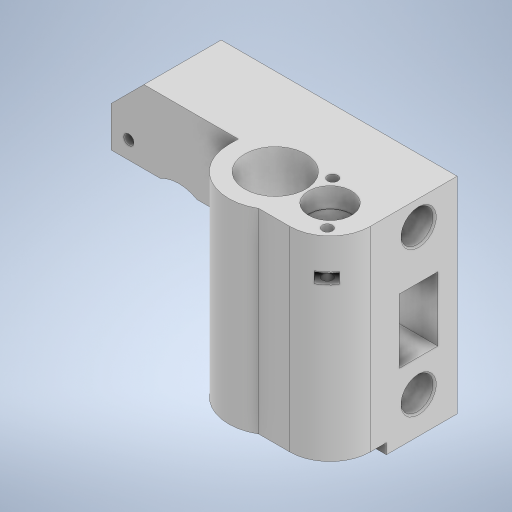
# Autodesk Inventor part: X-End-motor v0.3
Saved by Autodesk Inventor 2023 (Build 270158000, 158)
## iProperties
Created: 2023-07-24
Part Number: X-End-motor v0.3
Material: Generic
Document SubType Name: Modeling
Designer: Parker
Density: 1 g/cm^3
Appearance: Default
Author: Parker
Autodesk Inventor part; units mm, degrees
ref_plane "TopRodPlane" through (0, 22.5, 0) normal (0, 1, 0) x (-1, 0, 0)
ref_plane "BottomRodPlane" through (0, -22.5, 0) normal (0, 1, 0) x (-1, 0, 0)
ref_plane "Work Plane3" through (0, 0, 15) normal (0, 0, 1) x (1, 0, 0)
ref_plane "Work Plane4" through (-17, 0, 0) normal (1, 0, 0) x (0, 1, 0)
ref_plane "MotorZPlane" through (0, -2.5, 0) normal (0, 1, 0) x (-1, 0, 0)
ref_plane "Work Plane6" through (-50, 0, 0) normal (1, 0, 0) x (0, 1, 0)
ref_plane "RearClearancePlane" through (0, 0, -14) normal (0, 0, 1) x (1, 0, 0)
ref_plane "RightClearancePlane" through (14.5, 0, 0) normal (1, 0, 0) x (0, 1, 0)
sketch "Z-Template" plane through (0, 0, 0) normal (0, 1, 0) x (-1, 0, 0)
  circle A0 centre (17, 15) radius 9.5
  circle A1 centre (0, 15) radius 4.5
  circle A2 centre (17, 15) radius 14.5
  line L0 (87.7, 0) -> (-29.2, 0) construction
  line L1 (-29.2, -14) -> (87.7, -14) construction
  circle A3 centre (0, 15) radius 12.5
  line L2 (-14.5, -22.7) -> (-14.5, 38.2) construction
  line L3 (71, 12) -> (-12.5, 12)
  line L4 (-12.5, 12) -> (-12.5, -12)
  line L5 (-12.5, -12) -> (71, -12)
  line L6 (71, -12) -> (71, 12)
  line L7 (71, 12) -> (-12.5, -12) construction
  line L8 (-12.5, 12) -> (71, -12) construction
  line L9 (50, 38.2) -> (50, -22.7) construction
  point P0 (0, 0)
  point P1 (29.25, 0)
  dimension "d7" = 19
  dimension "d8" = 9
  dimension "d9" = 5
  dimension "d11" = 25
  dimension "d12" = 2
  dimension "d13" = 2
  dimension "d14" = 21
  constraints: 12 end point, 4 centre point, 3 coincident, 3 midpoint, 2 parallel, 1 horizontal, 1 perpendicular
  measures "d7" diameter of A0
  measures "d8" diameter of A1
  measures "d9" radial gap between concentric circles of A0 A2
  measures "d11" diameter of A3
  measures "d12" distance between parallel lines of L2 L4
  measures "d13" distance between parallel lines of L1 L5
  measures "d14" distance between parallel lines of L6 L9
ref_plane "TopPlane" through (0, 30, 0) normal (0, 1, 0) x (-1, 0, 0)
sketch "X-Template" plane through (0, 0, 0) normal (0, 0, 1) x (1, 0, 0)
  line L0 (-71, 18.5) -> (-29, 18.5)
  line L1 (-29, 18.5) -> (-29, -23.5)
  line L2 (-29, -23.5) -> (-71, -23.5)
  line L3 (-71, -23.5) -> (-71, 18.5)
  line L4 (-71, 18.5) -> (-29, -23.5) construction
  line L5 (-29, 18.5) -> (-71, -23.5) construction
  line L6 (-65.5, 13) -> (-34.5, 13) construction
  line L7 (-34.5, 13) -> (-34.5, -18) construction
  line L8 (-34.5, -18) -> (-65.5, -18) construction
  line L9 (-65.5, -18) -> (-65.5, 13) construction
  line L10 (-65.5, 13) -> (-34.5, -18) construction
  line L11 (-34.5, 13) -> (-65.5, -18) construction
  circle A0 centre (-65.5, 13) radius 1.6
  circle A1 centre (-34.5, 13) radius 1.6
  circle A2 centre (-34.5, -18) radius 1.6
  circle A3 centre (-65.5, -18) radius 1.6
  circle A4 centre (-50, -2.5) radius 11.5
  line L12 (-87.7, 22.5) -> (29.2, 22.5) projected
  line L13 (-87.7, -22.5) -> (29.2, -22.5) projected
  line L14 (14.5, 42.75) -> (14.5, -46.5) projected
  line L15 (-87.7, 30) -> (29.2, 30) projected
  line L16 (-19, 15) -> (12.5, 15)
  line L17 (12.5, 15) -> (12.5, 30)
  line L18 (12.5, 30) -> (-19, 30)
  line L19 (-19, 30) -> (-19, 15)
  line L20 (-19, 15) -> (12.5, 30) construction
  line L21 (12.5, 15) -> (-19, 30) construction
  line L22 (-19, -30) -> (12.5, -30)
  line L23 (-19, -15) -> (-19, -30)
  line L24 (12.5, -15) -> (-19, -15)
  line L25 (12.5, -30) -> (12.5, -15)
  line L26 (-17, -46.5) -> (-17, 42.75) projected
  line L27 (-7.5, -30.5) -> (-26.5, -30.5)
  line L28 (-26.5, -30.5) -> (-26.5, 30) construction
  line L29 (-26.5, 30) -> (-7.5, 30)
  line L30 (-7.5, 30) -> (-7.5, -30.5) construction
  line L31 (-7.5, -30.5) -> (-26.5, 30) construction
  line L32 (-26.5, -30.5) -> (-7.5, 30) construction
  line L33 (-31.5, 30) -> (-2.5, 30)
  line L34 (-2.5, 30) -> (-2.5, -30.5)
  line L35 (-2.5, -30.5) -> (-31.5, -30.5)
  line L36 (-31.5, -30.5) -> (-31.5, 30)
  line L37 (-31.5, 30) -> (-2.5, -30.5) construction
  line L38 (-2.5, 30) -> (-31.5, -30.5) construction
  point P0 (0, 0)
  point P1 (-3.25, 22.5)
  point P2 (-17, -0.25)
  dimension "d16" = 42
  dimension "d17" = 42
  dimension "d18" = 31
  dimension "d19" = 31
  dimension "d20" = 3.2
  dimension "d21" = 3.2
  dimension "d22" = 3.2
  dimension "d23" = 3.2
  dimension "d24" = 23
  dimension "d25" = 0
  dimension "d26" = 2
  dimension "d27" = 31.5
  dimension "d30" = 45
  dimension "d35" = 60.5
  dimension "d36" = 19
  dimension "d37" = 29
  constraints: 68 end point, 10 midpoint, 10 parallel, 5 centre point, 5 coincident, 5 horizontal, 5 perpendicular, 4 point on line, 1 vertical, 8 other
  measures "d16" distance of L1.end L2.end
  measures "d17" distance of L0.end L1.end
  measures "d18" distance of L7.end L8.end
  measures "d19" distance of L6.end L7.end
  measures "d20" diameter of A0
  measures "d21" diameter of A1
  measures "d22" diameter of A2
  measures "d23" diameter of A3
  measures "d24" diameter of A4
  measures "d25" distance between parallel lines of L15 L18
  measures "d26" distance between parallel lines of L14 L17
  measures "d27" distance between parallel lines of L17 L19
  measures "d30" distance of L16.start L22.start
  measures "d35" distance of L27.end L28.end
  measures "d36" distance between parallel lines of L30 L28
  measures "d37" distance of L34.end L35.end
sketch "Y-Template" plane through (0, 0, 0) normal (1, 0, 0) x (0, 1, 0)
  line L0 (-2.5, 38.2) -> (-2.5, -22.7) construction
  circle A0 centre (22.5, 0) radius 5
  circle A1 centre (-22.5, 0) radius 5
  line L1 (-46.5, 0) -> (42.75, 0) construction
  line L2 (-46.5, 0) -> (42.75, 0) projected
  line L3 (7.5, 6) -> (-12.5, 6)
  line L4 (-12.5, 6) -> (-12.5, -6)
  line L5 (-12.5, -6) -> (7.5, -6)
  line L6 (7.5, -6) -> (7.5, 6)
  line L7 (7.5, 6) -> (-12.5, -6) construction
  line L8 (-12.5, 6) -> (7.5, -6) construction
  line L9 (30, 38.2) -> (30, -22.7) construction
  circle A2 centre (22.5, 0) radius 7.5
  circle A3 centre (-22.5, 0) radius 7.5
  line L10 (-46.5, -14) -> (42.75, -14) projected
  line L11 (-33.75, 29.5) -> (-33.75, -14)
  line L12 (-33.75, -14) -> (30, -14)
  line L13 (30, -14) -> (30, 29.5)
  line L14 (-33.75, 29.5) -> (30, 29.5)
  line L15 (-46.5, 15) -> (42.75, 15) projected
  point P0 (0, 0)
  point P1 (-2.5, 0)
  dimension "d38" = 10
  dimension "d39" = 10
  dimension "d40" = 20
  dimension "d41" = 12
  dimension "d42" = 2.5
  dimension "d43" = 2.5
  dimension "d44" = 11.25
  dimension "d45" = 0
  dimension "d46" = 14.5
  constraints: 20 end point, 4 centre point, 3 point on line, 2 coincident, 2 horizontal, 2 midpoint, 2 parallel, 2 perpendicular, 1 vertical, 3 other
  measures "d38" diameter of A0
  measures "d39" diameter of A1
  measures "d40" distance of L5.end L4.end
  measures "d41" distance of L4.end L3.end
  measures "d42" radial gap between concentric circles of A0 A2
  measures "d43" radial gap between concentric circles of A1 A3
  measures "d44" distance from line of point (-22.5, 0) L11
  measures "d45" distance between parallel lines of L10 L12
  measures "d46" distance between parallel lines of L15 L14
sketch "Z-Drawing" plane through (0, 0, 0) normal (0, 1, 0) x (-1, 0, 0)
  line L0 (71, 12) -> (-12.5, 12) construction
  line L1 (71, -12) -> (71, 12) construction
  line L2 (-12.5, -12) -> (71, -12) construction
  line L3 (-12.5, 12) -> (-12.5, -12) construction
  circle A0 centre (0, 15) radius 12.5 construction
  circle A1 centre (17, 15) radius 14.5 construction
  circle A2 centre (17, 15) radius 9.5 construction
  circle A3 centre (0, 15) radius 4.5 construction
  line L4 (-12.5, 12) -> (-12.5, 15)
  line L5 (0, 27.5) -> (9.6515, 27.5)
  line L6 (31.5, 15) -> (31.5, 12)
  arc A4 (31.5, 15) -> (9.6515, 27.5) centre (17, 15) ccw
  line L7 (31.5, 12) -> (71, 12)
  circle A5 centre (17, 15) radius 9.5
  circle A6 centre (0, 15) radius 4.5
  arc A7 (0, 27.5) -> (-12.5, 15) centre (0, 15) ccw
  line L8 (71, 12) -> (71, -12)
  line L9 (71, -12) -> (-12.5, -12)
  line L10 (-12.5, -12) -> (-12.5, 12)
  point P0 (0, 0)
  dimension "d47" = 19
  dimension "d48" = 9
  dimension "d49" = 0
  constraints: 14 end point, 8 point on circle, 4 centre point, 4 coincident, 3 perpendicular, 2 collinear, 2 tangent, 1 horizontal, 1 point on line
  measures "d47" diameter of A5
  measures "d48" diameter of A6
  measures "d49" horizontal distance of A0.centre L5.start
extrude "Extrusion1" add sketch "Z-Drawing" against normal blind 60.5 from surface at 30
sketch "Y-Sketch" plane through (0, 0, 0) normal (1, 0, 0) x (0, 1, 0)
  circle A0 centre (22.5, 0) radius 5 projected
  line L0 (-12.5, 6) -> (-12.5, -6) projected
  line L1 (-12.5, -6) -> (7.5, -6) projected
  line L2 (7.5, -6) -> (7.5, 6) projected
  line L3 (7.5, 6) -> (-12.5, 6) projected
  circle A1 centre (-22.5, 0) radius 5 projected
  point P0 (0, 0)
extrude "Extrusion2" cut sketch "Y-Sketch" along normal through all both and the other way through all contours L3 L2 L1 L0
extrude "Extrusion3" cut sketch "Y-Sketch" against normal blind 26.5 from surface at 12.5 contours A0 | A1
sketch "X-Sketch" plane through (0, 0, 0) normal (0, 0, 1) x (1, 0, 0)
  circle A0 centre (-65.5, 13) radius 1.6 projected
  circle A1 centre (-34.5, 13) radius 1.6 projected
  circle A2 centre (-34.5, -18) radius 1.6 projected
  circle A3 centre (-50, -2.5) radius 11.5 projected
  line L0 (-71, -30.5) -> (12.5, -30.5) projected
  line L1 (-71, -30.5) -> (-71, 30) projected
  line L2 (-71, 30) -> (12.5, 30) projected
  line L3 (12.5, -30.5) -> (12.5, 30) projected
  line L4 (-71, 7.5) -> (12.5, 7.5) projected
  line L5 (-71, -12.5) -> (-71, 7.5) projected
  line L6 (12.5, -12.5) -> (-71, -12.5) projected
  line L7 (12.5, 7.5) -> (12.5, -12.5) projected
  line L8 (-71, 18.5) -> (-29, 18.5) projected
  line L9 (-29, 18.5) -> (-29, -23.5) projected
  line L10 (-29, -23.5) -> (-71, -23.5) projected
  line L11 (-38.5, 7.5) -> (-38.5, -30.5)
  point P0 (0, 0)
  point P1 (-44.3211, 7.5)
  point P2 (-55.6789, 7.5)
  dimension "d56" = 11.5
  constraints: 2 end point, 2 point on line, 1 perpendicular
  measures "d56" distance from line of A3.centre L11
extrude "Extrusion4" cut sketch "X-Sketch" along normal through all both and the other way through all contours A3 L6 L4 | L11 L6 A3 | A3 L4 L11 | L4 A3 | L6 L11 L10 L1 A3 | A3 L6 | A3 L6 L1 L4 | L11 L0 L1 L10
hole "Hole1" at (-65.5, 13, 0) at (-34.5, 13, 0) at (-34.5, -18, 0) direction (0, 0, -1) diameter 3.2 end through all both
sketch "Sketch7" plane through (12.5, 30, -12) normal (0, 0, -1) x (-1, 0, 0)
  line L0 (84, -54) -> (41, -54)
  line L1 (41, -54) -> (41, -11)
  line L2 (41, -11) -> (84, -11)
  line L3 (84, -11) -> (84, -54)
  line L4 (84, -54) -> (41, -11) construction
  line L5 (41, -54) -> (84, -11) construction
  point P0 (12.5, -30)
  point P1 (62.5, -32.5)
  dimension "d66" = 43
  dimension "d67" = 43
  constraints: 12 end point, 2 midpoint, 2 parallel, 1 horizontal, 1 perpendicular
  measures "d66" distance of L1.end L2.end
  measures "d67" distance of L0.end L1.end
extrude "Extrusion5" cut sketch "Sketch7" against normal blind 1.5
chamfer "Chamfer1" distance 10 angle 45 1 edges at (-71, 30, 0)
sketch "Sketch8" plane through (-9.6515, -30.5, 27.5) normal (0, -1, 0) x (1, 0, 0)
  line L0 (22.1515, -39.5) -> (22.1515, -12.5) projected
  line L1 (22.1515, -39.5) -> (12.1515, -39.5)
  line L2 (12.1515, -39.5) -> (12.1515, -17.5)
  line L3 (12.1515, -17.5) -> (22.1515, -17.5)
  line L4 (22.1515, -17.5) -> (22.1515, -39.5)
  point P0 (9.6515, -27.5)
  point P1 (14.1515, -31.75)
  point P2 (17.1515, -39.5)
  point P3 (14.1515, -22.25)
  dimension "d73" = 7.75
  dimension "d74" = 8
  dimension "d75" = 10
  dimension "d76" = 9.5
  dimension "d77" = 22
  dimension "d78" = 8
  constraints: 8 end point, 2 parallel, 1 horizontal, 1 midpoint, 1 perpendicular
  measures "d73" vertical distance of point (17.152, -39.5) point (14.152, -31.75)
  measures "d74" distance from line of L0 point (14.152, -31.75)
  measures "d75" distance of L2.end L3.end
  measures "d76" distance of point (14.152, -31.75) point (14.152, -22.25)
  measures "d77" distance of L1.end L2.end
  measures "d78" distance from line of L0 point (14.152, -22.25)
extrude "Extrusion6" add sketch "Sketch8" along normal blind 3.25
sketch "Sketch9" plane through (-9.6515, -33.75, 27.5) normal (0, -1, 0) x (1, 0, 0)
  point P0 (9.6515, -27.5)
  point P1 (14.1515, -22.25)
  point P2 (14.1515, -31.75)
hole "Hole2" at (4.5, -33.75, 5.25) at (4.5, -33.75, -4.25) direction (0, 1, 0) diameter 1.8 depth 5
sketch "Sketch10" plane through (-9.6515, -30.5, 27.5) normal (0, -1, 0) x (1, 0, 0)
  line L0 (12.1515, -17.5) -> (22.1515, -17.5) projected
  line L1 (22.1515, -17.5) -> (22.1515, -12.5) projected
  arc A0 (22.1515, -12.5) -> (9.6515, 0) centre (9.6515, -12.5) ccw projected
  line L2 (9.6515, 0) -> (0, 0) projected
  arc A1 (0, 0) -> (-21.8485, -12.5) centre (-7.3485, -12.5) ccw projected
  line L3 (-21.8485, -12.5) -> (-21.8485, -15.5) projected
  line L4 (-21.8485, -15.5) -> (-28.8485, -15.5) projected
  line L5 (-28.8485, -15.5) -> (-28.8485, -39.5) projected
  line L6 (-28.8485, -39.5) -> (12.1515, -39.5) projected
  line L7 (12.1515, -39.5) -> (12.1515, -17.5) projected
  circle A2 centre (-7.3485, -12.5) radius 9.5 projected
  circle A3 centre (9.6515, -12.5) radius 4.5 projected
  line L8 (-16.8485, -3) -> (2.1515, -3)
  line L9 (2.1515, -3) -> (2.1515, -22)
  line L10 (2.1515, -22) -> (-16.8485, -22)
  line L11 (-16.8485, -22) -> (-16.8485, -3)
  line L12 (-16.8485, -3) -> (2.1515, -22) construction
  line L13 (2.1515, -3) -> (-16.8485, -22) construction
  line L14 (-14.3485, -3) -> (-0.3485, -3)
  line L15 (-0.3485, -3) -> (-0.3485, -22)
  line L16 (-0.3485, -22) -> (-14.3485, -22)
  line L17 (-14.3485, -22) -> (-14.3485, -3)
  line L18 (-14.3485, -3) -> (-0.3485, -22) construction
  line L19 (-0.3485, -3) -> (-14.3485, -22) construction
  point P0 (9.6515, -27.5)
  point P1 (-0.3485, -6.0774)
  point P2 (-0.3485, -18.9226)
  point P3 (-14.3485, -18.9226)
  point P4 (-14.3485, -6.0774)
  dimension "d88" = 19
  dimension "d89" = 19
  dimension "d90" = 14
  constraints: 24 end point, 4 midpoint, 4 parallel, 2 horizontal, 2 perpendicular, 1 point on line
  measures "d88" distance of L9.end L10.end
  measures "d89" distance of L8.end L9.end
  measures "d90" distance of L15.end L16.end
extrude "Extrusion7" add sketch "Sketch10" against normal blind 2.5 contours A2 L15 | L17 A2
sketch "Sketch11" plane through (0, 30, 0) normal (0, 1, 0) x (-1, 0, 0)
  circle A0 centre (0, 15) radius 4.5 projected
  line L0 (-6.2896, 22.1197) -> (6.2896, 7.8803)
  circle A1 centre (6.2896, 7.8803) radius 1.6
  circle A2 centre (-6.2896, 22.1197) radius 1.6
  line L1 (0, 27.5) -> (9.6515, 27.5) projected
  line L2 (0.0022, 23.8793) -> (0.0022, 18.3793) construction
  line L3 (-12.5, -12) -> (-12.5, 15) projected
  circle A3 centre (0, 15) radius 6.65
  line L4 (-0.7348, 6.8652) -> (2.1876, 2.0883)
  line L5 (2.1876, 2.0883) -> (13.3141, 8.8953)
  line L6 (13.3141, 8.8953) -> (10.3916, 13.6722)
  line L7 (10.3916, 13.6722) -> (-0.7348, 6.8652)
  line L8 (-0.7348, 6.8652) -> (13.3141, 8.8953) construction
  line L9 (2.1876, 2.0883) -> (10.3916, 13.6722) construction
  line L10 (10.1393, 6.953) -> (7.2169, 11.73)
  line L11 (7.2169, 11.73) -> (2.4399, 8.8075)
  line L12 (2.4399, 8.8075) -> (5.3624, 4.0306)
  line L13 (5.3624, 4.0306) -> (10.1393, 6.953)
  line L14 (10.1393, 6.953) -> (2.4399, 8.8075) construction
  line L15 (7.2169, 11.73) -> (5.3624, 4.0306) construction
  line L16 (-1.2297, 20.7298) -> (-5.3657, 16.9544)
  line L17 (-5.3657, 16.9544) -> (-11.3495, 23.5097)
  line L18 (-11.3495, 23.5097) -> (-7.2136, 27.2851)
  line L19 (-7.2136, 27.2851) -> (-1.2297, 20.7298)
  line L20 (-1.2297, 20.7298) -> (-11.3495, 23.5097) construction
  line L21 (-5.3657, 16.9544) -> (-7.2136, 27.2851) construction
  line L22 (-6.045, 26.072) -> (-10.2419, 22.3644)
  line L23 (-10.2419, 22.3644) -> (-6.5343, 18.1675)
  line L24 (-6.5343, 18.1675) -> (-2.3374, 21.8751)
  line L25 (-2.3374, 21.8751) -> (-6.045, 26.072)
  line L26 (-6.045, 26.072) -> (-6.5343, 18.1675) construction
  line L27 (-10.2419, 22.3644) -> (-2.3374, 21.8751) construction
  circle A4 centre (17, 15) radius 9.5 projected
  point P0 (0, 0)
  point P1 (-7.2582, 21.1293)
  point P2 (7.2582, 8.8707)
  point P3 (-6.5004, 18.1974)
  point P4 (-2.4454, 21.8463)
  point P5 (2.4399, 8.8075)
  point P6 (5.3624, 4.0306)
  point P7 (-8.373, 20.2489)
  point P8 (-6.0789, 26.042)
  point P9 (-4.2063, 23.9906)
  dimension "d98" = 19
  dimension "d99" = 3.2
  dimension "d100" = 3.2
  dimension "d102" = 5.5
  dimension "d105" = 13.3
  dimension "d106" = 5.6
  dimension "d107" = 5.6
  dimension "d108" = 5.6
  dimension "d109" = 5.6
  dimension "d110" = 5.6
  dimension "d111" = 5.6
  dimension "d112" = 100
  constraints: 52 end point, 9 midpoint, 8 parallel, 5 coincident, 4 perpendicular, 3 centre point, 1 point on line, 1 vertical
  measures "d98" distance of L0.start L0.end
  measures "d99" diameter of A1
  measures "d100" diameter of A2
  measures "d102" distance of L2.start L2.end
  measures "d105" diameter of A3
  measures "d106" distance of L4.start L4.end
  measures "d107" distance of L10.start L10.end
  measures "d108" distance of L11.end L10.end
  measures "d109" distance of L16.start L16.end
  measures "d110" distance of L22.start L22.end
  measures "d111" distance of L23.end L22.end
  measures "d112" angle of L0 L7
extrude "Extrusion8" cut sketch "Sketch11" against normal blind 6 contours A0 L0 | A0 L0 L16 L19 A3 | L0 A0 | A0 L0 A3 L7 L17 L16 | L16 L17 A3 L0 | L0 A3 L19 L16 | A3 L7
ref_plane "Work Plane10" through (0, 17, 0) normal (0, 1, 0) x (-1, 0, 0)
extrude "Extrusion10" cut sketch "Sketch11" against normal blind 18 contours A1 | A2
extrude "Extrusion11" cut sketch "Sketch11" along normal blind 2.5 from surface at -13 contours L16 L17 A3 L0 | L0 A3 L19 L16 | L7 L10 L5 L12 A3 | A3 L17 L24 L0 | L0 L24 L25 L19 A3 | A3 L7 | L7 A4 L5 L10 | L24 L17 L23 L22 L19 L25 | L7 L6 L5 A4 | L24 L23 L17 | L17 L18 L19 L22 L23 picked at (11.1512, 10.477)
chamfer "Chamfer2" distance 1 angle 45 1 edges at (-9.1721, 19.5, 9.6173)
chamfer "Chamfer3" distance 1 angle 45 1 edges at (8.3094, 19.5, 24.3383)
chamfer "Chamfer4" distance 2 angle 45 1 edges at (4.5, 24, 15)
chamfer "Chamfer5" distance 0.5 angle 45 2 edges at (12.5, 17.5, 0) (12.5, -27.5, 0)
chamfer "Chamfer6" distance 1.5 angle 45 1 edges at (-33.5, -24, -12)
move faces "Move1" translate (0, 0.2, 0) faces at (-22.215, 30, -6.1436)
equation "\"d30\" = X_Rod_Spacing"
equation "\"d54\" = Overlap"
equation "\"X_Rod_Spacing\" = 45"
equation "\"d0\" = 0.5 * X_Rod_Spacing"
equation "\"d1\" = -X_Rod_Spacing"
equation "\"Z_Rod_Forward_Offset\" = 15"
equation "\"d2\" = Z_Rod_Forward_Offset"
equation "\"Z_Drive_Offset\" = 17"
equation "\"d3\" = -Z_Drive_Offset"
equation "\"RearClearance\" = 14"
equation "\"d6\" = -RearClearance"
equation "\"RightClearance\" = 14.5"
equation "\"d10\" = RightClearance"
equation "\"Overlap\" = 26.5"
